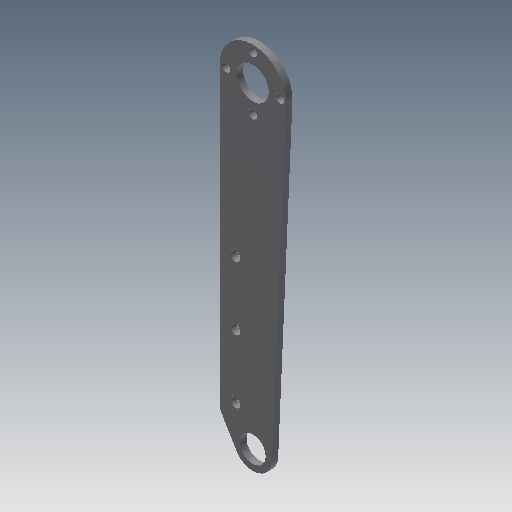
# Autodesk Inventor part: リンク_ふくらはぎ_メインフレーム_1_1
Saved by Autodesk Inventor 2017.3 (Build 213256000, 256)
## iProperties
Created: 2016-04-27
Part Number: リンク_ふくらはぎ_メインフレーム_1_1
Material: GFRP
Document SubType Name: Modeling
Designer: hiroaki
Density: 1.75 g/cm^3
Appearance: 滑らか - 淡い灰色
Mass: 6.71575 g
Surface Area: 45.847 cm^2
Volume: 3.83757 cm^3
d0: 1.000 ul
d2: 4.000 ul
d4: 360.00 deg
d6: 10.100 mm
d7: 12.000 mm
d8: 3.100 mm
d10: 5.000 mm
d11: 10.000 mm
d12: 4.000 mm
d13: 40.000 mm
d14: 2.000 mm
d15: 0.00 deg
Author: hiroaki
Autodesk Inventor part; units mm, degrees
ref_plane "YZ Plane" through (0, 0, 0) normal (1, 0, 0) x (0, 1, 0)
ref_plane "XZ Plane" through (0, 0, 0) normal (0, 1, 0) x (-1, 0, 0)
ref_plane "XY Plane" through (0, 0, 0) normal (0, 0, 1) x (1, 0, 0)
derived "下半身全体像_1_1.ipt"
sketch "スケッチ1" plane through (0, 0, 0) normal (0, 0, 1) x (1, 0, 0)
  circle A0 centre (0, 0) radius 10.5 construction
  line L0 (0, 0) -> (-12, 0) construction
  arc A1 (0, 16) -> (-12, 10.583) centre (0, 0) ccw construction
  arc A2 (-12, -10.583) -> (0, -16) centre (0, 0) ccw construction
  line L1 (0, 16) -> (39.5, 16) construction
  line L2 (39.5, 16) -> (39.5, -16) construction
  line L3 (39.5, -16) -> (0, -16) construction
  circle A3 centre (1, 13.5) radius 1.35
  circle A4 centre (1, -13.5) radius 1.35
  circle A5 centre (28, 13.5) radius 1.35
  circle A6 centre (28, -13.5) radius 1.35
  line L4 (1, 13.5) -> (1, -13.5) construction
  line L5 (1, -13.5) -> (28, -13.5) construction
  line L6 (1, 13.5) -> (28, 13.5) construction
  line L7 (28, 13.5) -> (28, -13.5) construction
  line L8 (0, 0) -> (1, 0) construction
  line L9 (32, 120) -> (32, 20) construction
  line L10 (0, 0) -> (0, 0) construction
  circle A7 centre (32, 120) radius 4.05
  line L11 (0, 140) -> (0, 40) construction
  circle A8 centre (0, 40) radius 4.05
  line L12 (0, 0) -> (0, -100) construction
  line L13 (32, 20) -> (32, -80) construction
  line L14 (0, 0) -> (0, 40) construction
  circle A9 centre (32, 20) radius 6.5 construction
  line L15 (32, 23.5218) -> (35.05, 21.7609) construction
  line L16 (35.05, 21.7609) -> (35.05, 18.2391) construction
  line L17 (35.05, 18.2391) -> (32, 16.4782) construction
  line L18 (32, 16.4782) -> (28.95, 18.2391) construction
  line L19 (28.95, 18.2391) -> (28.95, 21.7609) construction
  line L20 (28.95, 21.7609) -> (32, 23.5218) construction
  line L21 (21.5, 152) -> (61, 152) construction
  line L22 (61, 152) -> (61, 100.5) construction
  line L23 (61, 100.5) -> (21.5, 100.5) construction
  line L24 (21.5, 100.5) -> (21.5, 152) construction
  line L25 (21.5, 140) -> (61, 140) construction
  line L26 (16, 150.5) -> (66.5, 150.5) construction
  line L27 (66.5, 150.5) -> (66.5, 129.5) construction
  line L28 (66.5, 129.5) -> (16, 129.5) construction
  line L29 (16, 129.5) -> (16, 150.5) construction
  circle A10 centre (0, 140) radius 10.5 construction
  line L30 (-13.5, 139) -> (13.5, 139) construction
  line L31 (13.5, 139) -> (13.5, 112) construction
  line L32 (13.5, 112) -> (-13.5, 112) construction
  line L33 (-13.5, 112) -> (-13.5, 139) construction
  circle A11 centre (-13.5, 139) radius 1.35
  circle A12 centre (13.5, 139) radius 1.35
  circle A13 centre (-13.5, 112) radius 1.35
  circle A14 centre (13.5, 112) radius 1.35
  line L34 (-12, 10.583) -> (-12, -10.583) construction
  circle A15 centre (0, -100) radius 4.05
  circle A16 centre (32, -80) radius 4.05
  circle A17 centre (0, -100) radius 10.5 construction
  line L35 (32, -80) -> (0, -100) construction
  line L36 (45, -60.5) -> (77.5, -60.5) construction
  line L37 (77.5, -60.5) -> (77.5, -112) construction
  line L38 (77.5, -112) -> (45, -112) construction
  line L39 (45, -112) -> (45, -60.5) construction
  line L40 (45, -100) -> (77.5, -100) construction
  line L41 (39.5, -89.5) -> (83, -89.5) construction
  line L42 (83, -89.5) -> (83, -110.5) construction
  line L43 (83, -110.5) -> (39.5, -110.5) construction
  line L44 (39.5, -110.5) -> (39.5, -89.5) construction
  line L45 (1, -86.5) -> (28, -86.5) construction
  line L46 (28, -86.5) -> (28, -113.5) construction
  line L47 (28, -113.5) -> (1, -113.5) construction
  line L48 (1, -113.5) -> (1, -86.5) construction
  circle A18 centre (1, -86.5) radius 1.35
  circle A19 centre (1, -113.5) radius 1.35
  circle A20 centre (28, -113.5) radius 1.35
  circle A21 centre (28, -86.5) radius 1.35
  circle A22 centre (32, 20) radius 4.05
  circle A23 centre (32, 20) radius 4.05
  line L49 (10.583, 152) -> (-10.583, 152) construction
  line L50 (16, 140) -> (16, 100.5) construction
  line L51 (16, 100.5) -> (-16, 100.5) construction
  line L52 (-16, 100.5) -> (-16, 140) construction
  arc A24 (16, 140) -> (10.583, 152) centre (0, 140) ccw construction
  arc A25 (-10.583, 152) -> (-16, 140) centre (0, 140) ccw construction
  line L53 (-12, -89.417) -> (-12, -110.583) construction
  line L54 (0, -84) -> (39.5, -84) construction
  line L55 (39.5, -84) -> (39.5, -116) construction
  line L56 (39.5, -116) -> (0, -116) construction
  arc A26 (0, -84) -> (-12, -89.417) centre (0, -100) ccw construction
  arc A27 (-12, -110.583) -> (0, -116) centre (0, -100) ccw construction
  circle A28 centre (0, 148.5) radius 1.35
  circle A29 centre (-8.5, 0) radius 1.35
  circle A30 centre (0, 0) radius 8.5 construction
  circle A31 centre (0, 140) radius 8.5 construction
  circle A32 centre (-8.5, 140) radius 1.35
  circle A33 centre (0, 131.5) radius 1.35
  circle A34 centre (8.5, 140) radius 1.35
  circle A35 centre (0, 140) radius 5.05
  circle A36 centre (0, 40) radius 6 construction
  circle A37 centre (-5.5, 90) radius 1.55
  circle A38 centre (-5.5, 70) radius 1.55
  circle A39 centre (-5.5, 50) radius 1.55
  line L57 (-5.5, 90) -> (-5.5, 50) construction
  line L58 (10.4894, 139.5275) -> (5.9939, 39.73)
  arc A40 (10.4894, 139.5275) -> (-10.5, 140) centre (0, 140) ccw
  arc A41 (-5.1692, 36.9538) -> (5.9939, 39.73) centre (0, 40) ccw
  line L59 (-5.1692, 36.9538) -> (-10.5, 46)
  line L60 (-10.5, 46) -> (-10.5, 94)
  line L61 (-10.5, 94) -> (-10.5, 140)
  line L62 (-5.5, 70) -> (-10.5, 70) construction
  line L63 (-5.5, 50) -> (6.4565, 50) construction
  circle A42 centre (-5.5, 50) radius 5 construction
  line L64 (-5.5, 50) -> (-10.5, 50) construction
  circle A43 centre (-5.5, 90) radius 5 construction
  line L65 (-5.5, 90) -> (-10.5, 90) construction
  line L66 (35.05, 121.7609) -> (35.05, 118.2391) construction
  line L67 (35.05, 118.2391) -> (32, 116.4782) construction
  line L68 (32, 116.4782) -> (28.95, 118.2391) construction
  line L69 (28.95, 118.2391) -> (28.95, 121.7609) construction
  line L70 (28.95, 121.7609) -> (32, 123.5218) construction
  line L71 (32, 123.5218) -> (35.05, 121.7609) construction
  line L72 (0, 152) -> (0, 140) construction
  line L73 (0, 140) -> (0, 139) construction
  point P0 (66.5, 140)
  point P1 (39.5, 0)
  point P2 (83, -100)
  point P3 (1, -100)
  point P4 (-12, -100)
  point P5 (39.5, -100)
  dimension "d4" = 360
  dimension "d6" = 10.1
  dimension "d7" = 12
  dimension "d8" = 3.1
  dimension "d10" = 5
  dimension "d11" = 10
  dimension "d12" = 4
  dimension "d13" = 40
  measures "d6" diameter of A35
  measures "d7" diameter of A36
  measures "d8" diameter of A37
  measures "d10" distance between parallel lines of L60 L57
  measures "d11" distance from line of L14.end L63
  measures "d12" distance from line of L59.end L64
  measures "d13" distance of L57.end L57.start
extrude "押し出し1" add sketch "スケッチ1" along normal blind 2 contours L58 A41 L59 L60 L61 A40
